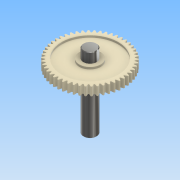
# Autodesk Inventor part: Редукторная  шестерня
Saved by Autodesk Inventor 2017 (Build 210142000, 142)
## iProperties
Part Number: Редукторная  шестерня
Material: Типовые
Document SubType Name: Modeling
Designer: STALKER
Density: 1 g/cm^3
Appearance: Светло-бежевый
Author: STALKER
Autodesk Inventor part; units mm, degrees
ref_plane "YZ Plane" through (0, 0, 0) normal (1, 0, 0) x (0, 1, 0)
ref_plane "XZ Plane" through (0, 0, 0) normal (0, 1, 0) x (-1, 0, 0)
sketch "Эскиз1" plane through (0, 0, 0) normal (0, 0, 1) x (1, 0, 0)
  circle A0 centre (0, 0) radius 2.5
  circle A1 centre (0, 0) radius 4
  circle A2 centre (0, 0) radius 10.6
  circle A3 centre (0, 0) radius 13
  line L0 (0, 0) -> (0, 17) construction
  line L1 (0, 0) -> (-21, 0) construction
  circle A4 centre (0, 0) radius 6
  dimension "d0" = 5
  dimension "d3" = 8
  dimension "d4" = 21.2
  dimension "d5" = 26
  dimension "d6" = 12
  constraints: 5 centre point, 5 coincident, 4 end point
  measures "d0" diameter of A0
  measures "d3" diameter of A1
  measures "d4" diameter of A2
  measures "d5" diameter of A3
  measures "d6" diameter of A4
extrude "Выдавливание1" add sketch "Эскиз1" along normal blind 3.7 contours A0
extrude "Выдавливание2" add sketch "Эскиз1" against normal blind 7 contours A1
extrude "Выдавливание3" add sketch "Эскиз1" against normal blind 7 contours A4
extrude "Выдавливание4" cut sketch "Эскиз1" against normal blind 0.8 contours A4
extrude "Выдавливание5" add sketch "Эскиз1" against normal blind 3.2 contours A3
extrude "Выдавливание6" add sketch "Эскиз1" against normal blind 2.4 contours A2
extrude "Выдавливание7" cut sketch "Эскиз1" against normal blind 0.8 contours A2
extrude "Выдавливание8" add sketch "Эскиз1" against normal blind 24.3 contours A0
chamfer "Фаска1" distance 0.2 angle 45 1 edges at (-6, 0, -7)
chamfer "Фаска2" distance 0.2 angle 45 1 edges at (-2.5, 0, 3.7)
ref_plane "РабПлоскость1" through (0, 0, -17.3) normal (0, 0, -1) x (-1, 0, 0)
chamfer "Фаска3" distance 0.2 angle 45 1 edges at (-2.5, 0, -24.3)
sketch "Эскиз3" plane through (0, 0, -3.2) normal (0, 0, -1) x (-1, 0, 0)
  arc A0 (12.9615, -0.2) -> (12.9615, 0.2) centre (0, 0) ccw
  circle A1 centre (0, 0) radius 11.9
  line L0 (0, 0) -> (20, 0) construction
  line L1 (0, 0) -> (0, 19) construction
  line L2 (12.9615, 0.2) -> (11.8849, 0.6)
  line L3 (12.9615, -0.2) -> (11.8849, -0.6)
  circle A2 centre (0, 0) radius 22.8035
  dimension "d35" = 23.8
  dimension "d36" = 0.4
  dimension "d37" = 1.2
  constraints: 8 end point, 4 point on circle, 3 centre point, 3 coincident, 1 horizontal, 1 other
  measures "d35" diameter of A1
  measures "d36" distance of L3.start L2.start
  measures "d37" distance of L3.end L2.end
extrude "Выдавливание10" cut sketch "Эскиз3" against normal blind 6
fillet "Сопряжение1" radius 0.1 4 edges at (-11.8849, -0.6, -1.6) (-11.8849, 0.6, -1.6) (-12.9615, -0.2, -1.6) (-12.9615, 0.2, -1.6)
pattern_circular "Круговой массив1" count 50 over 360 about axis through (0, 0, 0) along (0, 0, -1)
sketch "Эскиз2" plane through (0, 0, -17.3) normal (0, 0, -1) x (-1, 0, 0)
  circle A0 centre (0, 0) radius 2.5
  line L0 (2, 1.5) -> (2, -1.5)
  dimension "d28" = 5
  dimension "d29" = 4.5
  constraints: 2 end point, 2 point on circle, 1 centre point, 1 coincident, 1 vertical
  measures "d28" diameter of A0
extrude "Выдавливание9" cut sketch "Эскиз2" against normal blind 6 contours A0 L0 picked at (2.0912, -0.3466)
